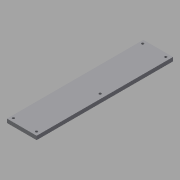
# Autodesk Inventor part: Top Plate
Saved by Autodesk Inventor 2013 (Build 170138000, 138)
## iProperties
Created: 2013-01-27
Part Number: Top Plate
Material: Aluminum 6061
Document SubType Name: Modeling
Designer: Naphat
Density: 1 g/cm^3
Author: Naphat
Autodesk Inventor part; units mm, degrees
ref_plane "YZ Plane" through (0, 0, 0) normal (1, 0, 0) x (0, 1, 0)
ref_plane "XZ Plane" through (0, 0, 0) normal (0, 1, 0) x (-1, 0, 0)
ref_plane "XY Plane" through (0, 0, 0) normal (0, 0, 1) x (1, 0, 0)
sketch "Sketch1" plane through (0, 0, 0) normal (0, 1, 0) x (-1, 0, 0)
  line L0 (0, 0) -> (-78.2, 0)
  line L1 (-78.2, 0) -> (-78.2, -359.6)
  line L2 (-78.2, -359.6) -> (0, -359.6)
  line L3 (0, -359.6) -> (0, 0)
  dimension "d0" = 78.2
  dimension "d1" = 359.6
  constraints: 8 end point, 2 perpendicular, 1 horizontal, 1 parallel
  measures "d0" distance of L0.start L0.end
  measures "d1" distance of L0.end L1.end
extrude "Extrusion1" add sketch "Sketch1" along normal blind 10
sketch "Sketch2" plane through (0, 0, 0) normal (0, -1, 0) x (1, 0, 0)
  circle A0 centre (7.62, -350.1) radius 3.175
  circle A1 centre (68.58, -350.1) radius 3.175
  circle A2 centre (7.62, -9.5) radius 3.175
  circle A3 centre (68.58, -9.5) radius 3.175
  constraints: 4 centre point
extrude "Extrusion2" cut sketch "Sketch2" against normal blind 25.4
sketch "Sketch3" plane through (0, 0, 0) normal (0, -1, 0) x (1, 0, 0)
  circle A0 centre (65.9, -179.8) radius 3.175
  dimension "d8" = 6.35
  constraints: 1 centre point
  measures "d8" diameter of A0
extrude "Extrusion3" cut sketch "Sketch3" against normal blind 25.4
body "Solid1"
